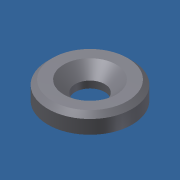
# Autodesk Inventor part: ARRUELA ESPECIAL DAS RODAS(31)
Saved by Autodesk Inventor 2012 SP1 (Build 160190100, 190)
## iProperties
Created: 2012-07-24
Part Number: ARRUELA ESPECIAL DAS RODAS(31)
Material: Carbon Steel
Document SubType Name: Modeling
Designer: bruno.silveira
Mass: 8.4619 g
Surface Area: 7.70083 cm^2
Volume: 1.07521 cm^3
Density: 7.87 g/cm^3
Author: bruno.silveira
Autodesk Inventor part; units mm, degrees
ref_plane "YZ Plane" through (0, 0, 0) normal (1, 0, 0) x (0, 1, 0)
ref_plane "XZ Plane" through (0, 0, 0) normal (0, 1, 0) x (-1, 0, 0)
ref_plane "XY Plane" through (0, 0, 0) normal (0, 0, 1) x (1, 0, 0)
sketch "Sketch1" plane through (0, 0, 0) normal (0, 0, 1) x (1, 0, 0)
  circle A0 centre (0, 0) radius 9.25
  dimension "d0" = 18.5
  constraints: 1 centre point, 1 coincident
  measures "d0" diameter of A0
extrude "Extrusion1" add sketch "Sketch1" along normal blind 4
sketch "Sketch2" plane through (0, 0, 4) normal (0, 0, 1) x (1, 0, 0)
  circle A0 centre (0, 0) radius 9.25 projected
hole "Hole1" at (0, 0, 4) direction (0, 0, -1) diameter 6.5 depth 4 tip angle 118 countersink diameter 11.5 countersink angle 90
chamfer "Chamfer1" distance 1 angle 45 1 edges at (-9.25, 0, 4)
body "Solid1"
